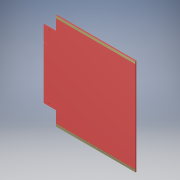
# Autodesk Inventor part: PayloadGermination_PCB
Saved by Autodesk Inventor 2018 (Build 220112000, 112)
## iProperties
Created: 2018-01-15
Part Number: PayloadGermination_PCB
Material: Epoxy Resin
Document SubType Name: Modeling
Designer: Bradley
Density: 1.14 g/cm^3
Appearance: Smooth - Red
Mass: 9.57888 g
Surface Area: 171.891 cm^2
Volume: 8.40253 cm^3
Author: Bradley
Revision Number: 3
Autodesk Inventor part; units mm, degrees
ref_plane "YZ Plane" through (0, 0, 0) normal (1, 0, 0) x (0, 1, 0)
ref_plane "XZ Plane" through (0, 0, 0) normal (0, 1, 0) x (-1, 0, 0)
ref_plane "XY Plane" through (0, 0, 0) normal (0, 0, 1) x (1, 0, 0)
sketch "Sketch1" plane through (0, 0, 0) normal (0, 0, 1) x (1, 0, 0)
  line L0 (0, 33.8) -> (12.5, 33.8)
  line L1 (12.5, 33.8) -> (12.5, 47.9)
  line L2 (12.5, 47.9) -> (91.4, 47.9)
  line L3 (91.4, 47.9) -> (91.4, -47.9)
  line L4 (91.4, -47.9) -> (12.5, -47.9)
  line L5 (12.5, -47.9) -> (12.5, -33.8)
  line L6 (12.5, -33.8) -> (0, -33.8)
  line L7 (0, -33.8) -> (0, 33.8)
  line L8 (-4.5, 48) -> (91.5, 48) construction
  line L9 (91.5, 48) -> (91.5, -48) construction
  line L10 (91.5, -48) -> (-4.5, -48) construction
  line L11 (-4.5, -48) -> (-4.5, 48) construction
  line L12 (-4.4, 47.9) -> (-3.4, 47.9) construction
  line L13 (-3.4, 47.9) -> (-3.4, -47.9) construction
  line L14 (-3.4, -47.9) -> (-4.4, -47.9) construction
  line L15 (-4.4, -47.9) -> (-4.4, 47.9) construction
  point P0 (0, 0)
  point P1 (0, 0)
  point P2 (-4.5, 0)
  dimension "d0" = 67.6
  dimension "d1" = 95.8
  dimension "d2" = 91.4
  dimension "d3" = 12.5
  dimension "d20" = 96
  dimension "d21" = 96
  dimension "d22" = 0.1
  dimension "d23" = 0.1
  dimension "d24" = 1
  dimension "d25" = 0.1
  dimension "d26" = 3.4
  constraints: 32 end point, 8 perpendicular, 4 parallel, 3 collinear, 3 horizontal, 2 midpoint, 2 point on line, 1 coincident, 1 horizontal alignment
  measures "d0" distance of L6.end L0.start
  measures "d1" distance of L2.end L3.end
  measures "d2" distance between parallel lines of L7 L3
  measures "d3" distance of L0.start L0.end
  measures "d20" distance of L8.start L8.end
  measures "d21" distance of L10.end L8.start
  measures "d22" distance between parallel lines of L2 L8
  measures "d23" distance between parallel lines of L9 L3
  measures "d24" distance between parallel lines of L15 L13
  measures "d25" distance between parallel lines of L15 L11
  measures "d26" distance between parallel lines of L7 L13
extrude "Extrusion1" add sketch "Sketch1" along normal mid plane 1
sketch "Sketch2" plane through (0, 0, 0.5) normal (0, 0, 1) x (1, 0, 0)
  line L0 (12.5, 33.8) -> (0, 33.8) projected
  line L1 (0, 33.8) -> (0, -33.8) projected
  line L2 (0, -33.8) -> (12.5, -33.8) projected
  line L3 (12.5, -33.8) -> (12.5, -47.9) projected
  line L4 (12.5, -47.9) -> (91.4, -47.9) projected
  line L5 (91.4, -47.9) -> (91.4, 47.9) projected
  line L6 (91.4, 47.9) -> (12.5, 47.9) projected
  line L7 (12.5, 47.9) -> (12.5, 33.8) projected
  line L8 (91.4, -47.9) -> (91.4, 47.9) projected
  line L9 (12.5, 47.9) -> (91.4, 47.9)
  line L10 (91.4, 47.9) -> (91.4, 45.4)
  line L11 (91.4, 45.4) -> (12.5, 45.4)
  line L12 (12.5, 45.4) -> (12.5, 47.9)
  line L13 (91.4, -47.9) -> (12.5, -47.9)
  line L14 (12.5, -47.9) -> (12.5, -45.4)
  line L15 (12.5, -45.4) -> (91.4, -45.4)
  line L16 (91.4, -45.4) -> (91.4, -47.9)
  point P0 (0, 0)
  dimension "d6" = 2.5
  dimension "d27" = 90.8
  constraints: 16 end point, 4 parallel, 2 horizontal, 2 perpendicular, 2 point on line, 1 collinear
  measures "d6" distance between parallel lines of L4 L15
  measures "d27" distance between parallel lines of L15 L11
extrude "Extrusion2" add sketch "Sketch2" along normal blind 0.01 contours L7 L6 L5 L11 | L5 L4 L3 L15
mirror "Mirror1" about plane through (0, 0, 0) normal (0, 0, 1) of "Extrusion2"
sketch "Sketch3" plane through (0, 0, 0.5) normal (0, 0, 1) x (1, 0, 0)
  circle A0 centre (6, 31.8) radius 0.9
  circle A1 centre (6, -31.8) radius 0.9
  point P0 (0, 0)
  dimension "d9" = 1.8
  dimension "d10" = 6
  dimension "d11" = 31.8
  dimension "d12" = 31.8
  constraints: 2 centre point, 1 equal radius, 1 vertical alignment
  measures "d9" diameter of A0
  measures "d10" horizontal distance of point (0, 0) A0.centre
  measures "d11" vertical distance of point (0, 0) A0.centre
  measures "d12" vertical distance of A1.centre point (0, 0)
extrude "Extrusion3" cut sketch "Sketch3" against normal through all
sketch "Sketch4" plane through (0, 0, 0.5) normal (0, 0, 1) x (1, 0, 0)
  circle A0 centre (6, 31.8) radius 0.9 projected
  circle A1 centre (6, -31.8) radius 0.9 projected
  line L0 (12.5, -45.4) -> (91.4, -45.4) projected
  line L1 (91.4, -45.4) -> (91.4, 45.4) projected
  line L2 (91.4, 45.4) -> (12.5, 45.4) projected
  line L3 (12.5, 45.4) -> (12.5, 33.8) projected
  line L4 (12.5, 33.8) -> (0, 33.8) projected
  line L5 (0, 33.8) -> (0, -33.8) projected
  line L6 (0, -33.8) -> (12.5, -33.8) projected
  line L7 (12.5, -33.8) -> (12.5, -45.4) projected
  line L8 (0, 18.95) -> (3.5, 18.95)
  arc A2 (3.5, 17.95) -> (3.5, 18.95) centre (3.5, 18.45) ccw
  line L9 (3.5, 17.95) -> (0, 17.95)
  point P0 (0, 0)
  dimension "d15" = 17.95
  dimension "d16" = 3.5
  dimension "d17" = 1
  constraints: 4 end point, 2 point on circle, 2 point on line, 2 tangent, 1 centre point, 1 horizontal, 1 perpendicular
  measures "d15" distance from line of point (0, 0) L9
  measures "d16" distance from line of A2.centre L5
  measures "d17" distance between parallel lines of L9 L8
extrude "Extrusion4" cut sketch "Sketch4" against normal through all contours L5 L8 A2 L9
equation "\"d23\" = d22"
equation "\"d25\" = d22"
equation "\"d12\" = d11"
body "Solid1"
